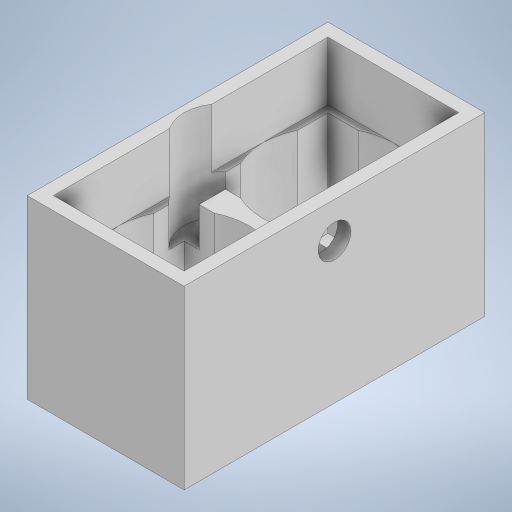
# Autodesk Inventor part: Suporte Eletroimã
Saved by Autodesk Inventor 2023 (Build 270158000, 158)
## iProperties
Created: 2023-03-07
Part Number: Suporte Eletroimã
Material: Genérico
Document SubType Name: Modeling
Designer: Inteli
Density: 1 g/cm^3
Appearance: Padrão
Author: Inteli
Autodesk Inventor part; units mm, degrees
ref_plane "YZ Plane" through (0, 0, 0) normal (1, 0, 0) x (0, 1, 0)
ref_plane "XZ Plane" through (0, 0, 0) normal (0, 1, 0) x (-1, 0, 0)
ref_plane "XY Plane" through (0, 0, 0) normal (0, 0, 1) x (1, 0, 0)
sketch "Esboço1" plane through (0, 0, 0) normal (0, 1, 0) x (-1, 0, 0)
  circle A0 centre (0, 11) radius 10
  circle A1 centre (0, -11) radius 10
  line L0 (9, 2) -> (-9, 2)
  line L1 (-9, -2) -> (9, -2)
  line L2 (9, 20) -> (-9, 20)
  line L3 (-9, -20) -> (9, -20)
  line L4 (12, 23) -> (-12, 23)
  line L5 (-12, 23) -> (-12, -23)
  line L6 (-12, -23) -> (12, -23)
  line L7 (12, -23) -> (12, 23)
  line L8 (9, -20) -> (9, -2)
  line L9 (9, 2) -> (9, 20)
  line L10 (-9, 20) -> (-9, 2)
  line L11 (-9, -2) -> (-9, -20)
  point P0 (-9, 6.6411)
  point P1 (-9, 15.3589)
  point P2 (-4.3589, 20)
  point P3 (4.3589, 20)
  point P4 (9, 15.3589)
  point P5 (9, 6.6411)
  point P6 (4.3589, 2)
  point P7 (-4.3589, 2)
  point P8 (-9, -6.6411)
  point P9 (-4.3589, -2)
  point P10 (4.3589, -2)
  point P11 (9, -6.6411)
  point P12 (9, -15.3589)
  point P13 (4.3589, -20)
  point P14 (-4.3589, -20)
  point P15 (-9, -15.3589)
  point P16 (0, 0)
  point P17 (0, 21)
  point P18 (0, 21)
  dimension "d16" = 40
  dimension "d17" = 18
  dimension "d18" = 24
  dimension "d61" = 46
  dimension "d62" = 22
  constraints: 24 end point, 8 parallel, 3 horizontal, 3 perpendicular, 2 coincident, 1 centre point, 3 other
  measures "d16" distance of L3.start L2.end
  measures "d17" distance of L3.start L3.end
  measures "d18" distance of L6.end L5.end
  measures "d61" distance of L4.end L5.end
  measures "d62" distance of point (0, 11) A1.centre
extrude "Base Principal dos Imãs" add sketch "Esboço1" along normal blind 25
sketch "Esboço9" plane through (0, 0, 0) normal (0, -1, 0) x (1, 0, 0)
  line L0 (-12, 23) -> (12, 23) projected
  line L1 (12, -23) -> (-12, -23) projected
  line L2 (12, 23) -> (-12, 23)
  line L3 (-12, 23) -> (-12, -23)
  line L4 (-12, -23) -> (12, -23)
  line L5 (12, -23) -> (12, 23)
  point P0 (0, 0)
  point P1 (12, -23)
  constraints: 8 end point, 2 parallel, 1 horizontal, 1 perpendicular
extrude "Fundo" add sketch "Esboço9" along normal blind 2
sketch "Esboço13" plane through (0, 25, 0) normal (0, 1, 0) x (1, 0, 0)
  line L0 (10, 21) -> (-10, 21)
  line L1 (-10, 21) -> (-10, -21)
  line L2 (-10, -21) -> (10, -21)
  line L3 (10, -21) -> (10, 21)
  line L4 (10, 21) -> (-10, -21) construction
  line L5 (-10, 21) -> (10, -21) construction
  point P0 (0, 0)
  dimension "d84" = 20
  dimension "d85" = 42
  constraints: 12 end point, 2 midpoint, 2 parallel, 1 horizontal, 1 perpendicular
  measures "d84" distance of L2.end L1.end
  measures "d85" distance of L1.end L0.end
extrude "PCB / Tampa" cut sketch "Esboço13" against normal blind 9
sketch "Esboço14" plane through (0, 25, 0) normal (0, 1, 0) x (1, 0, 0)
  line L0 (-9, -2) -> (-4.3589, -2) projected
  line L1 (-6.6794, -2) -> (-9, -4.3206)
  line L2 (-9, -6.6411) -> (-9, -2) projected
  line L3 (-6.6794, -2) -> (-6.6794, 2)
  line L4 (-9, 2) -> (-4.3589, 2) projected
  line L5 (-9, 2) -> (-9, 6.6411) projected
  line L6 (-9, 4.3206) -> (-6.6794, 2)
  arc A0 (-9, 4.3206) -> (-9, -4.3206) centre (-5.3332, 0) ccw
  point P0 (0, 0)
  constraints: 6 end point, 4 midpoint, 2 point on circle, 1 centre point, 1 perpendicular
extrude "Espaço Fio (Validar)" cut sketch "Esboço14" against normal blind 15
sketch "Esboço15" plane through (10, 25, -21) normal (-1, 0, 0) x (0, 0, 1)
  circle A0 centre (21, -5.5) radius 2.5
  point P0 (21, -25)
  dimension "d90" = 5
  constraints: 1 centre point
  measures "d90" diameter of A0
extrude "Extrusão14" cut sketch "Esboço15" against normal up to surface (2 mm away)
